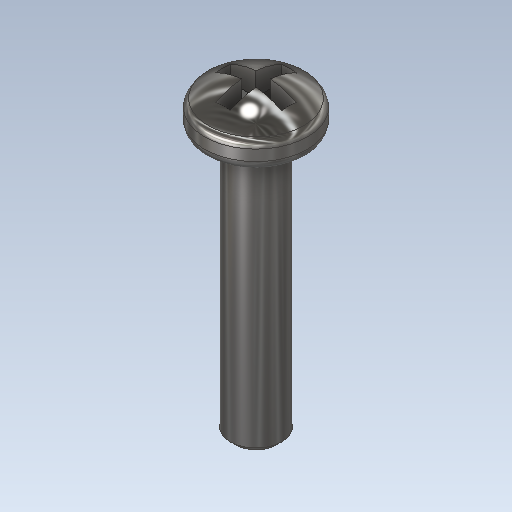
# Autodesk Inventor part: pan_head_screw
Saved by Autodesk Inventor 2020.1 (Build 241239000, 239)
## iProperties
Created: 2018-11-23
Part Number: pan_head_screw
Material: Stainless Steel, Polished
Document SubType Name: Modeling
Designer: Petar
Density: 8 g/cm^3
Appearance: Stainless - Polished
Mass: 5.84896 g
Surface Area: 6.80218 cm^2
Volume: 0.73112 cm^3
Author: Petar
Autodesk Inventor part; units mm, degrees
ref_plane "YZ Plane" through (0, 0, 0) normal (1, 0, 0) x (0, 1, 0)
ref_plane "XZ Plane" through (0, 0, 0) normal (0, 1, 0) x (-1, 0, 0)
sketch "Sketch1" plane through (0, 0, 0) normal (0, 0, 1) x (1, 0, 0)
  line L0 (0, 0) -> (0, 25.4)
  line L1 (2.5, 25.4) -> (2.5, 0)
  line L2 (2.5, 0) -> (0, 0)
  line L3 (0, 25.4) -> (0, 29.9)
  arc A0 (5, 27.9) -> (0, 29.9) centre (0, 22.65) ccw
  line L4 (2.5, 25.4) -> (5, 25.4)
  line L5 (-9.3694, 47.064) -> (8.7897, 47.064) construction
  line L6 (8.7897, 47.064) -> (8.7897, -18.3846) construction
  line L7 (8.7897, -18.3846) -> (-9.3694, -18.3846) construction
  line L8 (-9.3694, -18.3846) -> (-9.3694, 47.064) construction
  line L9 (5, 25.4) -> (5, 27.9)
  dimension "d0" = 25.4
  dimension "d1" = 2.5
  dimension "d2" = 4.5
  dimension "d4" = 2.5
  dimension "d31" = 2.5
  dimension "d33" = 2.5
  constraints: 12 end point, 3 vertical, 2 point on circle, 1 centre point, 1 horizontal, 1 line through centre, 1 parallel, 1 perpendicular, 2 other
  measures "d0" distance of L0.start L0.end
  measures "d1" distance of L0.end L1.start
  measures "d2" distance of L0.end L3.end
  measures "d4" distance of L4.end L1.start
  measures "d31" distance of L4.end L9.end
  measures "d33" distance from line of L0 L1.start
revolve "Revolution1" add sketch "Sketch1" angle 360 about axis through (0, 0, 0) along (0, 1, 0)
chamfer "Chamfer1" distance 0.5 angle 45 1 edges at (-2.5, 0, 0)
fillet "Fillet1" radius 1 2 edges at (-5, 25.4, 0) (-5, 27.9, 0)
ref_plane "Work Plane1" through (0, 29.9, 0) normal (0, -1, 0) x (1, 0, 0)
sketch "Sketch4" plane through (0, 29.9, 0) normal (0, -1, 0) x (1, 0, 0)
  line L0 (0.7, 0.7) -> (0.7, 3.2)
  line L1 (0.7, 3.2) -> (-0.7, 3.2)
  line L2 (-0.7, 3.2) -> (-0.7, 0.7)
  line L3 (0.7, 0.7) -> (3.2, 0.7)
  line L4 (3.2, 0.7) -> (3.2, -0.7)
  line L5 (3.2, -0.7) -> (0.7, -0.7)
  line L6 (0.7, -0.7) -> (0.7, -3.2)
  line L7 (0.7, -3.2) -> (-0.7, -3.2)
  line L8 (-0.7, -3.2) -> (-0.7, -0.7)
  line L9 (-0.7, -0.7) -> (-3.2, -0.7)
  line L10 (-3.2, -0.7) -> (-3.2, 0.7)
  line L11 (-3.2, 0.7) -> (-0.7, 0.7)
  point P0 (0, 0)
  dimension "d57" = 2.5
  dimension "d58" = 1.4
  dimension "d59" = 2.5
  dimension "d60" = 1.4
  dimension "d61" = 2.5
  dimension "d62" = 2.5
  dimension "d63" = 1.4
  dimension "d64" = 90
  dimension "d65" = 2.5
  dimension "d66" = 1.4
  dimension "d67" = 90
  constraints: 24 end point, 7 perpendicular, 5 point on line, 1 vertical
  measures "d57" distance of L0.start L0.end
  measures "d58" distance of L0.end L1.end
  measures "d59" distance of L0.start L3.end
  measures "d60" distance of L3.end L4.end
  measures "d61" distance of L4.end L5.end
  measures "d62" distance of L5.end L6.end
  measures "d63" distance of L6.end L7.end
  measures "d64" angle of L6 L7
  measures "d65" distance of L8.end L9.end
  measures "d66" distance of L9.end L10.end
  measures "d67" angle of L9 L10
extrude "Extrusion1" cut sketch "Sketch4" along normal blind 3
chamfer "Chamfer2" distance 0.7 angle 45 12 edges at (0.7, 26.9, -1.95) (0, 26.9, -3.2) (-0.7, 26.9, -1.95) (-1.95, 26.9, -0.7) (-3.2, 26.9, 0) (-1.95, 26.9, 0.7) (-0.7, 26.9, 1.95) (1.95, 26.9, -0.7) (3.2, 26.9, 0) (1.95, 26.9, 0.7) (0.7, 26.9, 1.95) (0, 26.9, 3.2)
body "Solid1"
